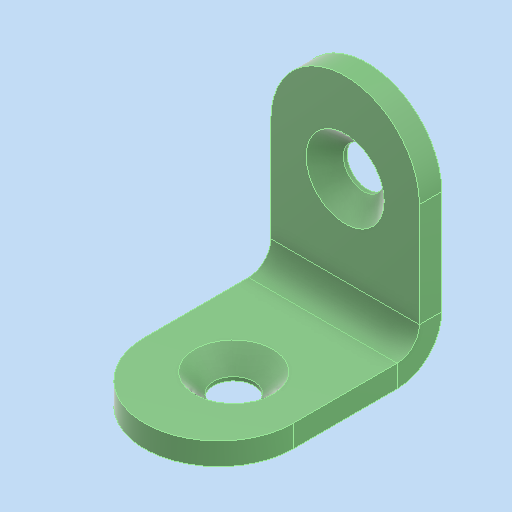
# Autodesk Inventor part: скоба
Saved by Autodesk Inventor 2025 (Build 290162000, 162)
## iProperties
Created: 2025-03-04
Part Number: скоба
Material: Типовые
Document SubType Name: Sheet Metal
Designer: volko
Density: 1 g/cm^3
Sheet Metal Rule: По умолчанию_мм
Appearance: По умолчанию
Author: volko
Autodesk Inventor part; units mm, degrees
ref_plane "YZ Plane" through (0, 0, 0) normal (1, 0, 0) x (0, 1, 0)
ref_plane "XZ Plane" through (0, 0, 0) normal (0, 1, 0) x (-1, 0, 0)
ref_plane "XY Plane" through (0, 0, 0) normal (0, 0, 1) x (1, 0, 0)
sketch "Эскиз1" plane through (0, 0, 0) normal (0, 0, 1) x (1, 0, 0)
  line L0 (-10, 0) -> (10, 0)
  line L1 (10, 0) -> (10, 20)
  line L2 (0, 30) -> (0, 30)
  line L3 (-10, 20) -> (-10, 0)
  arc A0 (0, 30) -> (-10, 20) centre (0, 20) ccw
  arc A1 (10, 20) -> (0, 30) centre (0, 20) ccw
  line L4 (0, -6.4142) -> (0, 38.4853)
  point P0 (0, 0)
  point P1 (0, 30)
  dimension "d0" = 20
  dimension "d1" = 10
  dimension "d2" = 20
  measures "d0" distance between parallel lines of L1 L3
  measures "d1" radius of A0
  measures "d2" distance of L0.end L1.end
extrude "Пластина1" add sketch "Эскиз1" along normal blind 3
sketch "Эскиз2" plane through (10, 3, 0) normal (0, -1, 0) x (1, 0, 0)
  line L0 (-20, 0) -> (0, 0)
  line L1 (0, 0) -> (0, 30)
  line L2 (0, 30) -> (-20, 30)
  line L3 (-20, 30) -> (-20, 0)
  constraints: 6 end point, 1 horizontal, 1 perpendicular, 1 vertical
edge flange "Фланец1" height 30 angle 90 thickness 3 bend radius 3 thickness toward (0, -1, 0) relief straight relief width 3 relief depth 1.5 edges at (0, 0, 3) wall of the first edge with corners at (-10, 3, 0) (10, 3, 0) (10, 3, 30) (-10, 3, 30)
bend "Сгиб1"
corner "УглСтык1"
fillet "Сопряжение1" radius 10 2 edges at (10, 1.5, 30) (-10, 1.5, 30)
sketch "Эскиз3" plane through (0, 0, 3) normal (0, 0, 1) x (1, 0, 0)
  line L0 (0, -6) -> (0, 36) projected
  arc A0 (10, 20) -> (-10, 20) centre (0, 20) ccw projected
  point P0 (0, 0)
  point P1 (0, 18)
  point P2 (0, 30)
  dimension "d29" = 12
  constraints: 1 point on circle, 1 point on line
  measures "d29" distance of point (0, 30) point (0, 18)
hole "Отверстие1" at (0, 18, 3) direction (0, 0, -1) diameter 5.5 end through all countersink diameter 10.5 countersink angle 90
sketch "Эскиз4" plane through (-10, 3, 6) normal (0, 1, 0) x (1, 0, 0)
  line L0 (0, 0) -> (0, -14) projected
  arc A0 (0, -14) -> (20, -14) centre (10, -14) ccw projected
  point P0 (10, 6)
  point P1 (10, -12)
  point P2 (10, -24)
  dimension "d30" = 10
  dimension "d31" = 12
  constraints: 1 point on circle
  measures "d30" distance from line of point (10, -12) L0
  measures "d31" distance of point (10, -12) point (10, -24)
hole "Отверстие2" at (0, 3, 18) direction (0, -1, 0) diameter 5.5 end through all countersink diameter 10.5 countersink angle 90
equation "\"d20\" = Толщина"
equation "\"d3\" = Толщина"
equation "\"d4\" = Ширина_просечки"
equation "\"d5\" = Глубина_просечки"
equation "\"d6\" = Мин_остаток"
equation "\"d7\" = Радиус_перехода"
equation "\"d10\" = Радиус_гибки"
equation "\"d11\" = Размер_просечки"
equation "\"d12\" = Размер_зазора"
equation "\"d13\" = Радиус_Якоби"
equation "\"Радиус_гибки\" = Толщина"
equation "\"Ширина_просечки\" = Толщина"
equation "\"Глубина_просечки\" = 0.5 * Толщина"
equation "\"Размер_просечки\" = 4 * Толщина"
equation "\"Мин_остаток\" = 2 * Толщина"
equation "\"Радиус_перехода\" = Радиус_гибки"
equation "\"Радиус_Якоби\" = Радиус_гибки"
equation "\"Размер_зазора\" = Толщина"
equation "\"Толщина\" = 3"
